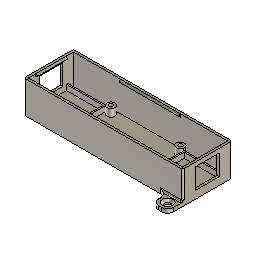
flexispot-passthrough-esp-case (Autodesk Fusion 360 design; units mm, degrees)
Autodesk Fusion 360 part; units mm, degrees
sketch "Skizze2" plane through (0, 0, 0) normal (0, 0, 1) x (1, 0, 0)
  line L0 (-50, -50) -> (53, -50)
  line L1 (53, -50) -> (53, -80)
  line L2 (53, -80) -> (-50, -80)
  line L3 (-50, -80) -> (-50, -50)
  line L4 (53, -65) -> (-50, -65) construction
  line L5 (-50, -54.8) -> (-25.84, -54.8)
  line L6 (-25.84, -54.8) -> (-25.84, -75.2)
  line L7 (-25.84, -75.2) -> (-50, -75.2)
  line L8 (-50, -75.2) -> (-50, -54.8)
  line L9 (-50, -54.6) -> (-25.64, -54.6)
  line L10 (-25.64, -54.6) -> (-25.64, -75.4)
  line L11 (-25.64, -75.4) -> (-50, -75.4)
  line L12 (-50, -53.6) -> (-24.64, -53.6)
  line L13 (-24.64, -53.6) -> (-24.64, -76.4)
  line L14 (-24.64, -76.4) -> (-50, -76.4)
  line L15 (1.5, -50) -> (1.5, -80)
  line L16 (28.84, -75.2) -> (53, -75.2)
  line L17 (53, -75.2) -> (53, -54.8)
  line L18 (28.84, -54.8) -> (28.84, -75.2)
  line L19 (53, -54.8) -> (28.84, -54.8)
  line L20 (28.64, -54.6) -> (28.64, -75.4)
  line L21 (28.64, -75.4) -> (53, -75.4)
  line L22 (53, -54.6) -> (28.64, -54.6)
  line L23 (27.64, -53.6) -> (27.64, -76.4)
  line L24 (27.64, -76.4) -> (53, -76.4)
  line L25 (53, -53.6) -> (27.64, -53.6)
  line L26 (-24.2111, -50.91) -> (27.3989, -50.91)
  line L27 (27.3989, -50.91) -> (27.3989, -79.36)
  line L28 (27.3989, -79.36) -> (-24.2111, -79.36)
  line L29 (-24.2111, -79.36) -> (-24.2111, -50.91)
  circle A0 centre (24.7989, -53.27) radius 1.5
  line L30 (24.7989, -53.27) -> (24.7989, -51.77) construction
  line L31 (24.7989, -51.77) -> (26.2989, -51.77) construction
  line L32 (26.2989, -51.77) -> (26.2989, -53.27) construction
  circle A1 centre (24.7989, -77) radius 1.5
  circle A2 centre (-21.6111, -77) radius 1.5
  circle A3 centre (-21.6111, -53.27) radius 1.5
  line L33 (24.7989, -77) -> (24.7989, -78.5) construction
  line L34 (26.2989, -78.5) -> (26.2989, -77) construction
  line L35 (-21.6111, -77) -> (-21.6111, -78.5) construction
  line L36 (-23.1111, -78.5) -> (-23.1111, -77) construction
  line L37 (-21.6111, -53.27) -> (-23.1111, -53.27) construction
  line L38 (-23.1111, -51.77) -> (-21.6111, -51.77) construction
  line L39 (-23.1111, -53.27) -> (-23.1111, -51.77) construction
  line L40 (54.5, -81.5) -> (-51.5, -81.5)
  line L41 (-51.5, -81.5) -> (-51.5, -48.5)
  line L42 (-51.5, -48.5) -> (54.5, -48.5)
  line L43 (54.5, -48.5) -> (54.5, -81.5)
  line L44 (-51.5, -48.5) -> (-41.5, -48.5)
  line L45 (-41.5, -48.5) -> (-41.5, -42.5)
  line L46 (-45.5, -38.5) -> (-47.5, -38.5)
  line L47 (-51.5, -42.5) -> (-51.5, -48.5)
  line L48 (54.5, -81.5) -> (44.5, -81.5)
  line L49 (44.5, -81.5) -> (44.5, -87.5)
  line L50 (48.5, -91.5) -> (50.5, -91.5)
  line L51 (54.5, -87.5) -> (54.5, -81.5)
  circle A4 centre (49.5, -86.5) radius 3
  circle A5 centre (-46.5, -43.5) radius 3
  arc A6 (-47.5, -38.5) -> (-51.5, -42.5) centre (-47.5, -42.5) ccw
  arc A7 (-41.5, -42.5) -> (-45.5, -38.5) centre (-45.5, -42.5) ccw
  arc A8 (44.5, -87.5) -> (48.5, -91.5) centre (48.5, -87.5) ccw
  arc A9 (50.5, -91.5) -> (54.5, -87.5) centre (50.5, -87.5) ccw
  circle A10 centre (-21.6111, -53.27) radius 2.7
  circle A11 centre (-21.6111, -77) radius 2.7
  circle A12 centre (24.7989, -77) radius 2.7
  circle A13 centre (24.7989, -53.27) radius 2.7
  point P0 (-51.5, -38.5)
  point P1 (54.5, -91.5)
  dimension "d1859" = 103
  dimension "d1860" = 30
  dimension "d1861" = 24.16
  dimension "d1862" = 20.4
  dimension "d1866" = 10.2
  dimension "d1867" = -0.2
  dimension "d1868" = -1.2
  dimension "d1869" = 51.61
  dimension "d1870" = 28.45
  dimension "d1873" = 3
  dimension "d1874" = 0.86
  dimension "d1875" = 1.1
  dimension "d1876" = 3
  dimension "d1877" = 3
  dimension "d1878" = 3
  dimension "d1879" = 0.86
  dimension "d1880" = 1.1
  dimension "d1881" = 1.1
  dimension "d1882" = 0.86
  dimension "d1883" = 0.86
  dimension "d1884" = 1.1
  dimension "d1886" = -1.5
  dimension "d1887" = 10
  dimension "d1888" = 10
  dimension "d1889" = 10
  dimension "d1890" = 10
  dimension "d1891" = 6
  dimension "d1892" = 6
  dimension "d1893" = 4
  dimension "d1904" = 1.2
  dimension "d1905" = 1.2
  dimension "d1906" = 1.2
  dimension "d1907" = 1.2
  constraint horizontal L0
  constraint vertical L1
  constraint horizontal L2
  constraint vertical L3
  constraint midpoint L1 L4.start
  constraint midpoint L3 L4.end
  constraint horizontal L5
  constraint vertical L6
  constraint horizontal L7
  constraint vertical L8
  constraint coincident L3 L5.start
  constraint midpoint L0 L15.start
  constraint midpoint L2 L15.end
  constraint symmetric L5.start L15 L17.end
  constraint symmetric L5.end L15 L18.start
  constraint symmetric L6.end L15 L16.start
  constraint symmetric L7.end L15 L16.end
  constraint symmetric L9.start L15 L22.start
  constraint symmetric L9.end L15 L20.start
  constraint symmetric L10.end L15 L20.end
  constraint symmetric L11.end L15 L21.end
  constraint symmetric L12.start L15 L25.start
  constraint symmetric L12.end L15 L23.start
  constraint symmetric L13.end L15 L23.end
  constraint symmetric L14.end L15 L24.end
  constraint horizontal L26
  constraint vertical L27
  constraint horizontal L28
  constraint vertical L29
  constraint coincident A0.centre L30.start
  constraint coincident A0 L30.end
  constraint perpendicular L26 L30
  constraint perpendicular L30 L31
  constraint coincident A0 L32.end
  constraint tangent A0 L32
  constraint coincident A1.centre L33.start
  constraint coincident A1 L33.end
  constraint vertical L33
  constraint coincident A1 L34.end
  constraint tangent A1 L34
  constraint coincident A2.centre L35.start
  constraint coincident A2 L35.end
  constraint perpendicular L28 L35
  constraint coincident A2 L36.end
  constraint tangent A2 L36
  constraint coincident A3.centre L37.start
  constraint coincident A3 L37.end
  constraint perpendicular L36 L37
  constraint coincident A3 L38.end
  constraint tangent A3 L38
  constraint perpendicular L38 L39
  constraint horizontal L44
  constraint vertical L45
  constraint horizontal L46
  constraint vertical L47
  constraint horizontal L48
  constraint vertical L49
  constraint horizontal L50
  constraint vertical L51
  constraint coincident P0 L46
  constraint coincident P0 L47
  constraint tangent L46 A6
  constraint tangent L47 A6
  constraint tangent L45 A7
  constraint tangent L46 A7
  constraint equal A6 A7
  constraint tangent L49 A8
  constraint tangent L50 A8
  constraint equal A6 A8
  constraint coincident P1 L50
  constraint coincident P1 L51
  constraint tangent L50 A9
  constraint tangent L51 A9
  constraint equal A6 A9
  measures "d1859" distance of L0.start L0.end
  measures "d1860" distance of L0.start L2.end
  measures "d1861" distance of L5.start L5.end
  measures "d1862" distance of L5.start L7.end
  measures "d1866" distance of L4 L5
  measures "d1869" distance of L26.start L26.end
  measures "d1870" distance of L26.start L28.end
  measures "d1873" diameter of A0
  measures "d1874" distance of L26 L31
  measures "d1875" distance of L27 L32
  measures "d1876" diameter of A1
  measures "d1877" diameter of A2
  measures "d1878" diameter of A3
  measures "d1879" distance of L26 L38
  measures "d1880" distance of L29 L39
  measures "d1881" distance of L29 L36
  measures "d1882" distance of L28 L35.end
  measures "d1883" distance of L28 L33.end
  measures "d1884" distance of L27 L34
  measures "d1887" distance of L41.end L44.end
  measures "d1888" distance of L41.end P0
  measures "d1889" distance of L40.start L48.end
  measures "d1890" distance of L40.start P1
  measures "d1891" diameter of A4
  measures "d1892" diameter of A5
  measures "d1893" radius of A6
extrude "Extrusion2" add sketch "Skizze2" along normal blind 20 and the other way blind 1.5 contours L40 L41 L42 L43 L44 L48 makes body 1
extrude "Extrusion3" add sketch "Skizze2" against normal blind 1.5 contours L0 L2 L3 L12 L13 L14 L15 L26 L28 L29 A10 A11 | L0 L1 L2 L15 L23 L24 L25 L26 L27 L28 A12 A13 | L3 L9 L10 L11 L12 L13 L14 | L15 L26 L27 L28 A12 A13 | L15 L26 L28 L29 A10 A11 | L3 L5 L6 L7 L9 L10 L11 | L1 L20 L21 L22 L23 L24 L25 | L26 L29 A10 | L26 A10 | L26 A13 | L26 L27 A13 | L3 L5 L6 L7 L8 | L1 L16 L18 L19 L20 L21 L22 | L27 L28 A12 | L28 A12 | L28 A11 | L28 L29 A11 | L26 L29 A10 | L26 L27 A13 | L27 A13 | L1 L16 L17 L18 L19 | L27 L28 A12 | L27 A12 | L28 L29 A11 | L29 A10 | L29 A11 | A0 | A1 | A2 | A3 | L40 L48 L49 L50 L51 A8 A9 | L40 L41 L42 L43 L44 L48 | L42 L44 L45 L46 L47 A6 A7 | A4 | A5 bodies 1
extrude "Extrusion4" add sketch "Skizze2" along normal blind 3.6 contours L3 L9 L10 L11 L12 L13 L14 | L1 L20 L21 L22 L23 L24 L25 bodies 1
extrude "Extrusion5" add sketch "Skizze2" along normal blind 5 contours L26 L29 A10 | L26 A10 | L26 A13 | L26 L27 A13 | L27 L28 A12 | L28 A12 | L28 A11 | L28 L29 A11 | A0 | A1 | A2 | A3 picked at (-21.6485, -51.1981) picked at (24.8362, -51.1981) picked at (24.8362, -79.0719) picked at (-21.6485, -79.0719) bodies 1
extrude "Extrusion6" add sketch "Skizze2" along normal blind 1 contours L40 L48 L49 L50 L51 A8 A9 | L42 L44 L45 L46 L47 A6 A7 | A4 | A5 bodies 1
fillet "Abrundung1" radius 5 2 edges at (-41.5, -48.5, -0.25) (44.5, -81.5, -0.25) on bodies 1
sketch "Skizze4" plane through (0, 0, 5) normal (0, 0, 1) x (-1, 0, 0)
  arc A0 (24.2111, 77.728) -> (24.2111, 76.272) centre (21.6111, 77) ccw
  line L0 (24.2111, 76.272) -> (24.2111, 77.728)
  point P0 (-24.7989, 77)
  point P1 (-24.7989, 53.27)
  point P2 (21.6111, 53.27)
  point P3 (21.6111, 77)
hole "Bohrung1" at (-21.6111, -77, 5) at (24.7989, -77, 5) at (24.7989, -53.27, 5) at (-21.6111, -53.27, 5) direction (0, 0, -1) diameter 2.529 depth 5 tip angle 180 bodies 1
thread "Gewinde1" "ISO Metric profile 3.0 M3x0.5 M3x0.5 6H" thread offset 0 thread depth 7.4
sketch "Skizze5" plane through (53, 0, 0) normal (-1, 0, 0) x (0, -1, 0)
  line L0 (76.4, 3.6) -> (76.4, 0)
  line L1 (76.4, 0) -> (80, 0)
  line L2 (80, 0) -> (80, 20)
  line L3 (80, 20) -> (50, 20)
  line L4 (50, 20) -> (50, 0)
  line L5 (50, 0) -> (53.6, 0)
  line L6 (53.6, 0) -> (53.6, 3.6)
  line L7 (53.6, 3.6) -> (54.6, 3.6)
  line L8 (54.6, 3.6) -> (54.6, 0)
  line L9 (54.6, 0) -> (75.4, 0)
  line L10 (75.4, 0) -> (75.4, 3.6)
  line L11 (75.4, 3.6) -> (76.4, 3.6)
  line L12 (54.6, 3.6) -> (53.6, 3.6)
  line L13 (53.6, 3.6) -> (76.4, 3.6)
  line L14 (76.4, 3.6) -> (75.4, 3.6)
  line L15 (75.4, 3.6) -> (54.6, 3.6)
  line L16 (57.1, 17.3) -> (72.9, 17.3)
  line L17 (72.9, 17.3) -> (72.9, 3.6)
  line L18 (72.9, 3.6) -> (57.1, 3.6)
  line L19 (57.1, 3.6) -> (57.1, 17.3)
  line L20 (65, 0) -> (65, 20) construction
  point P0 (54.6, 0)
  point P1 (75.4, 3.6)
  point P2 (54.6, 3.6)
  dimension "d1917" = 15.8
  dimension "d1918" = 13.7
  dimension "d1919" = 7.9
  constraint horizontal L16
  constraint vertical L17
  constraint horizontal L18
  constraint vertical L19
  constraint midpoint L9 L20.start
  constraint midpoint L3 L20.end
  constraint collinear L15 L18
  measures "d1917" distance of L17 L19
  measures "d1918" distance of L16 L18
  measures "d1919" distance of L17 L20
extrude "Extrusion7" cut sketch "Skizze5" along normal blind 115.0958 and the other way blind 16.016 contours L13 L15 L16 L17 L18 L19 bodies 1
sketch "Skizze6" plane through (0, 0, 1) normal (0, 0, 1) x (-1, 0, 0)
  arc A0 (41.5, 42.5) -> (45.5, 38.5) centre (45.5, 42.5) ccw
  line L0 (45.5, 38.5) -> (47.5, 38.5)
  arc A1 (47.5, 38.5) -> (51.5, 42.5) centre (47.5, 42.5) ccw
  line L1 (51.5, 42.5) -> (51.5, 48.5)
  line L2 (51.5, 48.5) -> (36.5, 48.5)
  arc A2 (41.5, 43.5) -> (36.5, 48.5) centre (36.5, 43.5) ccw
  line L3 (41.5, 43.5) -> (41.5, 42.5)
  point P0 (46.5, 43.5)
  point P1 (-49.5, 86.5)
hole "Bohrung2" at (-46.5, -43.5, 1) at (49.5, -86.5, 1) direction (0, 0, -1) diameter 4 depth 6 tip angle 180 countersink diameter 7 countersink angle 90 bodies 1
sketch "Skizze7" plane through (0, 0, 20) normal (0, 0, 1) x (-1, 0, 0)
  line L0 (-53, 50) -> (-53, 80)
  line L1 (-53, 80) -> (50, 80)
  line L2 (50, 80) -> (50, 50)
  line L3 (50, 50) -> (-53, 50)
  line L4 (-54.5, 81.5) -> (-54.5, 48.5)
  line L5 (-54.5, 48.5) -> (51.5, 48.5)
  line L6 (51.5, 48.5) -> (51.5, 81.5)
  line L7 (51.5, 81.5) -> (-54.5, 81.5)
  line L8 (49.7, 50.3) -> (-52.7, 50.3)
  line L9 (-52.7, 50.3) -> (-52.7, 79.7)
  line L10 (-52.7, 79.7) -> (49.7, 79.7)
  line L11 (49.7, 79.7) -> (49.7, 50.3)
  line L12 (48.2, 51.8) -> (-51.2, 51.8)
  line L13 (-51.2, 51.8) -> (-51.2, 78.2)
  line L14 (-51.2, 78.2) -> (48.2, 78.2)
  line L15 (48.2, 78.2) -> (48.2, 51.8)
  dimension "d1929" = 0.3
  dimension "d1930" = 1.8
extrude "Extrusion8" add sketch "Skizze7" along normal blind 2 separate body contours L0 L1 L2 L3 | L4 L5 L6 L7 | L8 L9 L10 L11 | L12 L13 L14 L15 makes body 2
extrude "Extrusion9" add sketch "Skizze7" against normal blind 2 contours L8 L9 L10 L11 bodies 2
ref_plane "Arbeitsebene1" through (1.5, -65, 9.25) normal (-1, 0, 0) x (0, -1, 0)
ref_plane "Arbeitsebene2" through (1.5, -65, 9.25) normal (0, -1, 0) x (1, 0, 0)
sketch "Skizze8" plane through (0, -65, 0) normal (0, -1, 0) x (-1, 0, 0)
  line L0 (-53, -20) -> (50, -20)
  line L1 (50, -20) -> (-53, -20)
  line L2 (-54.5, -20) -> (51.5, -20)
  line L3 (51.5, -20) -> (-54.5, -20)
  line L4 (50, 0) -> (-53, 0)
  line L5 (-53, 0) -> (-53, -20)
  line L6 (-53, -20) -> (50, -20)
  line L7 (50, -20) -> (50, 0)
  line L8 (50, -20) -> (48.9393, -18.9393)
  line L9 (50, -20) -> (47.5, -20) construction
  line L10 (48.9393, -18.9393) -> (50, -17.8787)
  dimension "d1935" = 45
  dimension "d1936" = 1.5
  constraint horizontal L9
  constraint coincident L0.end L1.start
  constraint coincident L7 L10.end
  constraint perpendicular L8 L10
  measures "d1935" angle of L8 L9
  measures "d1936" distance of L0.end L8.end
sketch "Skizze9" plane through (1.5, 0, 0) normal (-1, 0, 0) x (0, -1, 0)
  line L0 (80, 0) -> (80, 20)
  line L1 (80, 20) -> (80, 0)
  line L2 (50, 20) -> (80, 20)
  line L3 (80, 20) -> (50, 20)
  line L4 (81.5, 20) -> (48.5, 20)
  line L5 (48.5, 20) -> (81.5, 20)
  line L6 (80, 20) -> (78.9393, 18.9393)
  line L7 (80, 20) -> (77.5, 20) construction
  line L8 (78.9393, 18.9393) -> (80.7071, 17.1716)
  dimension "d1937" = 45
  dimension "d1938" = 1.5
  dimension "d1939" = 2.5
  constraint horizontal L7
  constraint coincident L0.end L1.start
  constraint perpendicular L6 L8
  measures "d1937" angle of L6 L7
  measures "d1938" distance of L0.end L6.end
  measures "d1939" distance of L6.end L8.end
extrude "Extrusion10" add sketch "Skizze9" along normal mid plane 40 bodies 1
extrude "Extrusion11" add sketch "Skizze8" along normal mid plane 20 contours L7 L8 L10 bodies 1
mirror "Spiegeln1" about plane through (1.5, -65, 9.25) normal (-1, 0, 0) of "Extrusion11"
mirror "Spiegeln2" about plane through (1.5, -65, 9.25) normal (0, -1, 0) of "Extrusion10"
combine "Kombinieren1" operation cut target body 2 tool bodies 1 keep tools
fillet "Abrundung2" radius 1 8 edges at (54.5, -48.5, 21) (1.5, -48.5, 22) (54.5, -65, 22) (1.5, -81.5, 22) (54.5, -81.5, 21) (-51.5, -65, 22) (-51.5, -48.5, 21) (-51.5, -81.5, 21) on bodies 2
fillet "Abrundung3" radius 1 6 edges at (-51.5, -81.5, 9.25) (-51.5, -48.5, 10.5) (54.5, -81.5, 10.5) (54.5, -48.5, 9.25) (47, -81.5, 1) (-44, -48.5, 1) on bodies 1
sketch "Skizze10" plane through (0, 0, 22) normal (0, 0, 1) x (-1, 0, 0)
  line L0 (50.5, 49.5) -> (50.5, 80.5)
  line L1 (50.5, 80.5) -> (-53.5, 80.5)
  line L2 (-53.5, 80.5) -> (-53.5, 49.5)
  line L3 (-53.5, 49.5) -> (50.5, 49.5)
  line L4 (-6.94, 70.8209) -> (-51.0504, 70.7321) construction
  line L5 (-51.0504, 70.7321) -> (-51.0242, 57.7315) construction
  line L6 (-51.0242, 57.7315) -> (-6.9138, 57.8204) construction
  line L7 (-6.9138, 57.8204) -> (-6.94, 70.8209) construction
  line L8 (47, 70.8206) -> (0, 70.8206) construction
  line L9 (0, 70.8206) -> (0, 57.8206) construction
  line L10 (0, 57.8206) -> (47, 57.8206) construction
  line L11 (47, 57.8206) -> (47, 70.8206) construction
  line L12 (-53.5, 65) -> (50.5, 65)
  dimension "d1952" = 5
  dimension "d1954" = 5
  text T0 "Keypad→" font "Arial" height 5 align right middle in box 44.1105 x 13.0006 at (-6.94, 70.8209) x (-0.999998, -0.002014) y (0.002014, -0.999998) spacing 1
  text T1 "← Desk CTRL" font "Arial" height 5 align left middle in box 47 x 13 at (47, 70.8206) x (-1, 0) y (0, -1) spacing 1
  constraint midpoint L2 L12.start
  constraint midpoint L0 L12.end
extrude "Extrusion12" cut sketch "Skizze10" against normal blind 1.5 text T1 T0 bodies 2
hidden bodies 2
equation "d1919 = ( 15.8 / 2 ) * 1 mm"
equation "d1953 = 'Keypad→'"
equation "d1955 = '← Desk CTRL'"
named bodies: "flexispot-passthrough-body", "flexispot-passthrough-deckel"
